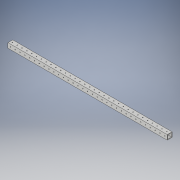
# Autodesk Inventor part: frame 2
Saved by Autodesk Inventor 2018 (Build 220112000, 112)
## iProperties
Created: 2018-02-01
Part Number: frame 2
Material: Generic
Document SubType Name: Modeling
Designer: cruz.anthony
Density: 1 g/cm^3
Appearance: Default
Author: cruz.anthony
Autodesk Inventor part; units mm, degrees
ref_plane "YZ Plane" through (0, 0, 0) normal (1, 0, 0) x (0, 1, 0)
ref_plane "XZ Plane" through (0, 0, 0) normal (0, 1, 0) x (-1, 0, 0)
ref_plane "XY Plane" through (0, 0, 0) normal (0, 0, 1) x (1, 0, 0)
sketch "Sketch1" plane through (0, 0, 0) normal (0, 1, 0) x (-1, 0, 0)
  line L0 (0, 0) -> (838.2, 0)
  line L1 (838.2, 0) -> (838.2, -25.4)
  line L2 (838.2, -25.4) -> (0, -25.4)
  line L3 (0, -25.4) -> (0, 0)
  dimension "d0" = 838.2
  dimension "d1" = 25.4
  constraints: 8 end point, 2 parallel, 1 horizontal, 1 perpendicular
  measures "d0" distance of L1.end L2.end
  measures "d1" distance of L0.end L1.end
extrude "Extrusion1" add sketch "Sketch1" along normal blind 25.4
sketch "Sketch2" plane through (0, 0, 0) normal (1, 0, 0) x (0, 0, -1)
  line L0 (3.175, 22.225) -> (22.225, 22.225)
  line L1 (22.225, 22.225) -> (22.225, 3.175)
  line L2 (22.225, 3.175) -> (3.175, 3.175)
  line L3 (3.175, 3.175) -> (3.175, 22.225)
  line L4 (0, 25.4) -> (25.4, 25.4) projected
  line L5 (0, 0) -> (0, 25.4) projected
  line L6 (25.4, 0) -> (0, 0) projected
  line L7 (25.4, 0) -> (25.4, 25.4) projected
  dimension "d4" = 3.175
  dimension "d5" = 3.175
  dimension "d6" = 3.175
  dimension "d7" = 3.175
  constraints: 8 end point, 2 parallel, 1 horizontal, 1 perpendicular
  measures "d4" distance between parallel lines of L4 L0
  measures "d5" distance between parallel lines of L5 L3
  measures "d6" distance between parallel lines of L6 L2
  measures "d7" distance between parallel lines of L7 L1
extrude "Extrusion2" cut sketch "Sketch2" against normal blind 838.2 contours L0 L1 L2 L3
sketch "Sketch4" plane through (-838.2, 0, 0) normal (0, 0, 1) x (1, 0, 0)
  circle A0 centre (825.5, 12.7) radius 1.9685
  line L0 (0, 25.4) -> (838.2, 25.4) projected
  line L1 (838.2, 0) -> (838.2, 25.4) projected
  circle A1 centre (800.1, 12.7) radius 1.9685
  circle A2 centre (774.7, 12.7) radius 1.9685
  circle A3 centre (749.3, 12.7) radius 1.9685
  circle A4 centre (723.9, 12.7) radius 1.9685
  circle A5 centre (698.5, 12.7) radius 1.9685
  circle A6 centre (673.1, 12.7) radius 1.9685
  circle A7 centre (647.7, 12.7) radius 1.9685
  circle A8 centre (622.3, 12.7) radius 1.9685
  circle A9 centre (596.9, 12.7) radius 1.9685
  circle A10 centre (571.5, 12.7) radius 1.9685
  circle A11 centre (546.1, 12.7) radius 1.9685
  circle A12 centre (520.7, 12.7) radius 1.9685
  circle A13 centre (495.3, 12.7) radius 1.9685
  circle A14 centre (469.9, 12.7) radius 1.9685
  circle A15 centre (444.5, 12.7) radius 1.9685
  circle A16 centre (419.1, 12.7) radius 1.9685
  circle A17 centre (393.7, 12.7) radius 1.9685
  circle A18 centre (368.3, 12.7) radius 1.9685
  circle A19 centre (342.9, 12.7) radius 1.9685
  circle A20 centre (317.5, 12.7) radius 1.9685
  circle A21 centre (292.1, 12.7) radius 1.9685
  circle A22 centre (266.7, 12.7) radius 1.9685
  circle A23 centre (241.3, 12.7) radius 1.9685
  circle A24 centre (215.9, 12.7) radius 1.9685
  circle A25 centre (190.5, 12.7) radius 1.9685
  circle A26 centre (165.1, 12.7) radius 1.9685
  circle A27 centre (139.7, 12.7) radius 1.9685
  circle A28 centre (114.3, 12.7) radius 1.9685
  circle A29 centre (88.9, 12.7) radius 1.9685
  circle A30 centre (63.5, 12.7) radius 1.9685
  circle A31 centre (38.1, 12.7) radius 1.9685
  circle A32 centre (12.7, 12.7) radius 1.9685
  dimension "d12" = 3.937
  dimension "d15" = 12.7
  dimension "d16" = 12.7
  dimension "d19" = 25.4
  dimension "d26" = 25.4
  dimension "d33" = 25.4
  dimension "d40" = 25.4
  constraints: 33 centre point, 4 horizontal, 64 other
  measures "d12" diameter of A0
  measures "d15" distance from line of L0 A0.centre
  measures "d16" distance from line of L1 A0.centre
  measures "d19" distance of A0.centre A1.centre
  measures "d26" distance of A11.centre A12.centre
  measures "d33" distance of A16.centre A17.centre
  measures "d40" distance of A27.centre A28.centre
extrude "Extrusion3" cut sketch "Sketch4" against normal blind 25.4
sketch "Sketch5" plane through (0, 25.4, 0) normal (0, 1, 0) x (1, 0, 0)
  circle A0 centre (-14.6685, 12.7) radius 1.9685
  line L0 (-838.2, 0) -> (0, 0) projected
  line L1 (0, 0) -> (0, 25.4) projected
  circle A1 centre (-40.0685, 12.7) radius 1.9685
  circle A2 centre (-65.4685, 12.7) radius 1.9685
  circle A3 centre (-90.8685, 12.7) radius 1.9685
  circle A4 centre (-116.2685, 12.7) radius 1.9685
  circle A5 centre (-141.6685, 12.7) radius 1.9685
  circle A6 centre (-167.0685, 12.7) radius 1.9685
  circle A7 centre (-192.4685, 12.7) radius 1.9685
  circle A8 centre (-217.8685, 12.7) radius 1.9685
  circle A9 centre (-243.2685, 12.7) radius 1.9685
  circle A10 centre (-268.6685, 12.7) radius 1.9685
  circle A11 centre (-294.0685, 12.7) radius 1.9685
  circle A12 centre (-319.4685, 12.7) radius 1.9685
  circle A13 centre (-344.8685, 12.7) radius 1.9685
  circle A14 centre (-370.2685, 12.7) radius 1.9685
  circle A15 centre (-395.6685, 12.7) radius 1.9685
  circle A16 centre (-421.0685, 12.7) radius 1.9685
  circle A17 centre (-446.4685, 12.7) radius 1.9685
  circle A18 centre (-471.8685, 12.7) radius 1.9685
  circle A19 centre (-497.2685, 12.7) radius 1.9685
  circle A20 centre (-522.6685, 12.7) radius 1.9685
  circle A21 centre (-548.0685, 12.7) radius 1.9685
  circle A22 centre (-573.4685, 12.7) radius 1.9685
  circle A23 centre (-598.8685, 12.7) radius 1.9685
  circle A24 centre (-624.2685, 12.7) radius 1.9685
  circle A25 centre (-649.6685, 12.7) radius 1.9685
  circle A26 centre (-675.0685, 12.7) radius 1.9685
  circle A27 centre (-700.4685, 12.7) radius 1.9685
  circle A28 centre (-725.8685, 12.7) radius 1.9685
  circle A29 centre (-751.2685, 12.7) radius 1.9685
  circle A30 centre (-776.6685, 12.7) radius 1.9685
  circle A31 centre (-802.0685, 12.7) radius 1.9685
  circle A32 centre (-827.4685, 12.7) radius 1.9685
  dimension "d47" = 3.937
  dimension "d48" = 12.7
  dimension "d49" = 12.7
  dimension "d52" = 25.4
  constraints: 33 centre point, 1 horizontal, 64 other
  measures "d47" diameter of A0
  measures "d48" distance from line of A0.centre L0
  measures "d49" distance edge to line of A0 L1
  measures "d52" distance of A0.centre A1.centre
extrude "Extrusion4" cut sketch "Sketch5" against normal blind 25.4
equation "\"d57\" = d52"
body "Solid1"
